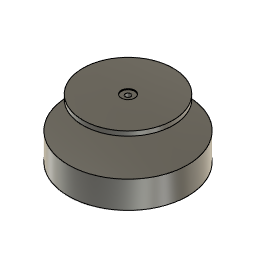
electroscope v7 (Autodesk Fusion 360 design; units mm, degrees)
Autodesk Fusion 360 part; units mm, degrees
sketch "bottle-mid" plane through (0, 0, 0) normal (0, 0, 1) x (1, 0, 0)
  circle A0 centre (0, 0) radius 27.5
  circle A1 centre (0, 0) radius 30.5
  circle A2 centre (0, 0) radius 33
  circle A3 centre (0, 0) radius 1.75
  circle A4 centre (0, 0) radius 24.25
  dimension "d19" = 55
  dimension "d20" = 3
  dimension "d21" = 5.5
  dimension "d34" = 3.5
  dimension "d37" = -3.25
  constraint coincident A0.centre A1.centre
  measures "d19" diameter of A0
  measures "d34" diameter of A3
extrude "Extrude7" add sketch "bottle-mid" against normal blind 15 contours A0 | A3 | A4 makes body 1
extrude "Extrude8" add sketch "bottle-mid" against normal blind 3 contours A1 bodies 1
extrude "Extrude9" add sketch "bottle-mid" against normal up to surface (15 mm away) contours A2 bodies 1
extrude "Extrude12" cut sketch "bottle-mid" against normal up to surface (15 mm away) contours A3 | A4 bodies 1
extrude "Extrude13" add sketch "bottle-mid" against normal blind 3 contours A4 bodies 1
sketch "top" plane through (0, 0, 0) normal (0, 0, 1) x (1, 0, 0)
  circle A0 centre (0, 0) radius 25
  circle A1 centre (0, 0) radius 3.75
  circle A2 centre (0, 0) radius 1.5
  dimension "d40" = 50
  dimension "d41" = 7.5
  dimension "d47" = 3
  constraint coincident A0.centre A1.centre
  measures "d40" diameter of A0
  measures "d41" diameter of A1
  measures "d47" diameter of A2
extrude "Extrude14" add sketch "top" along normal blind 15 separate body contours A1 | A2 makes body 2
extrude "Extrude15" add sketch "top" along normal blind 2.5 from surface at 15 contours A0 bodies 2
extrude "Extrude16" cut sketch "top" along normal up to surface (15 mm away) contours A2 bodies 2
extrude "Extrude17" add 1 faces at (2.9805, -0.2608, 15) along direction (0, 0, 1) blind 2 on bodies 2 bodies 2
named bodies: "bottle-mid", "collector"
